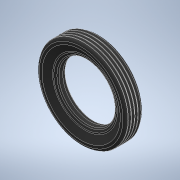
# Autodesk Inventor part: tire
Saved by Autodesk Inventor 2021 (Build 250183000, 183)
## iProperties
Created: 2022-05-13
Part Number: tire
Material: Generic
Document SubType Name: Modeling
Designer: kajet
Density: 1 g/cm^3
Appearance: Rubber - Black
Author: kajet
Autodesk Inventor part; units mm, degrees
ref_plane "YZ Plane" through (0, 0, 0) normal (1, 0, 0) x (0, 1, 0)
ref_plane "XZ Plane" through (0, 0, 0) normal (0, 1, 0) x (-1, 0, 0)
ref_plane "XY Plane" through (0, 0, 0) normal (0, 0, 1) x (1, 0, 0)
sketch "Sketch1" plane through (0, 0, 0) normal (0, 0, 1) x (1, 0, 0)
  circle A0 centre (0, 0) radius 175
  circle A1 centre (0, 0) radius 112.5 construction
  circle A2 centre (0, 0) radius 137.5
  dimension "d0" = 350
  dimension "d1" = 225
  dimension "d3" = 275
  constraints: 3 centre point, 3 coincident
  measures "d0" diameter of A0
  measures "d1" diameter of A1
  measures "d3" diameter of A2
sketch "Sketch2" plane through (0, 0, 0) normal (1, 0, 0) x (0, 1, 0)
  line L0 (175, 0) -> (-175, 0) projected
  line L1 (137.5, 0) -> (-137.5, 0) projected
  line L2 (165, 35) -> (0, 35)
  arc A0 (175, 25) -> (165, 35) centre (165, 25) ccw
  line L3 (175, 25) -> (176.5, 25)
  line L4 (175, 0) -> (175, 1.25)
  line L5 (175, 1.25) -> (176.5, 1.25)
  line L6 (176.5, 25) -> (176.5, 14.375)
  line L7 (176.5, 14.375) -> (175, 14.375)
  line L8 (175, 14.375) -> (175, 11.875)
  line L9 (175, 11.875) -> (176.5, 11.875)
  line L10 (176.5, 1.25) -> (176.5, 11.875)
  line L11 (176.5, 14.375) -> (176.5, 25)
  line L12 (175, 0) -> (175, 1.25)
  line L13 (175, 11.875) -> (175, 14.375)
  line L14 (165, 35) -> (154.375, 35)
  line L15 (112.5, 0) -> (-112.5, 0) construction
  line L16 (154.375, 35) -> (127.853, 19.6875)
  line L17 (154.375, 35) -> (185, 35) construction
  line L18 (127.853, 19.6875) -> (122.853, 19.6875)
  line L19 (112.5, 0) -> (107.5, 0)
  line L20 (122.853, 19.6875) -> (114.8887, 15.6007)
  arc A1 (110.6738, 11.4897) -> (107.5, 0) centre (133.6725, -1.0464) ccw
  arc A2 (114.8887, 15.6007) -> (110.6738, 11.4897) centre (119.4541, 6.7037) ccw
  line L21 (165, -35) -> (0, -35)
  arc A3 (165, -35) -> (175, -25) centre (165, -25) ccw
  line L22 (175, -25) -> (176.5, -25)
  line L23 (175, 0) -> (175, -1.25)
  line L24 (175, -1.25) -> (176.5, -1.25)
  line L25 (176.5, -25) -> (176.5, -14.375)
  line L26 (176.5, -14.375) -> (175, -14.375)
  line L27 (175, -14.375) -> (175, -11.875)
  line L28 (175, -11.875) -> (176.5, -11.875)
  line L29 (176.5, -1.25) -> (176.5, -11.875)
  line L30 (176.5, -14.375) -> (176.5, -25)
  line L31 (175, 0) -> (175, -1.25)
  line L32 (175, -11.875) -> (175, -14.375)
  line L33 (165, -35) -> (154.375, -35)
  line L34 (154.375, -35) -> (127.853, -19.6875)
  line L35 (154.375, -35) -> (185, -35) construction
  line L36 (127.853, -19.6875) -> (122.853, -19.6875)
  line L37 (122.853, -19.6875) -> (114.8887, -15.6007)
  arc A4 (107.5, 0) -> (110.6738, -11.4897) centre (133.6725, 1.0464) ccw
  arc A5 (110.6738, -11.4897) -> (114.8887, -15.6007) centre (119.4541, -6.7037) ccw
  line L38 (0, -51.8995) -> (0, 51.8995) projected
  point P0 (0, 0)
  point P1 (175, 35)
  point P2 (112.5, 14.375)
  point P3 (175, -35)
  point P4 (112.5, -14.375)
  dimension "d4" = 35
  dimension "d5" = 10
  dimension "d7" = 1.5
  dimension "d8" = 1.25
  dimension "d10" = 2.5
  dimension "d11" = 10.625
  dimension "d12" = 25
  dimension "d13" = 176.5
  dimension "d14" = 10.625
  dimension "d15" = 150
  dimension "d16" = 5
  dimension "d17" = 5
  dimension "d18" = 10
  constraints: 70 end point, 22 symmetric about line, 16 point on circle, 9 perpendicular, 7 point on line, 6 centre point, 5 tangent, 2 horizontal, 2 vertical, 1 equal length, 1 parallel, 3 other
  measures "d4" distance of L0.start point (175, 35)
  measures "d5" radius of A0
  measures "d7" distance of L3.start L3.end
  measures "d8" distance of L0.start L4.end
  measures "d10" distance of L7.end L8.end
  measures "d11" distance of L3.end L6.end
  measures "d12" distance of L0.start L3.start
  measures "d13" distance from line of point (0, 0) L10
  measures "d14" distance of L14.start L14.end
  measures "d15" angle of L16 L17
  measures "d16" distance of L16.end L18.end
  measures "d17" distance of L15.start L19.end
  measures "d18" radius of A2
revolve "Revolution1" add sketch "Sketch2" angle 360 about axis through (0, 0, -10) along (0, 0, 1) contours L23 L24 L29 L28 L27 L26 L25 L22 A3 L21 L34 L36 L37 A5 A4 L0 | L0 A1 A2 L20 L18 L16 L2 A0 L3 L6 L7 L8 L9 L10 L5 L4
body "Solid1"
